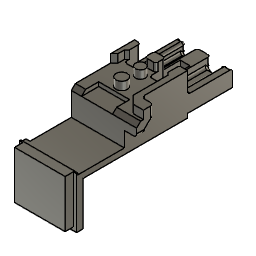
Sony PSP 1000 v29 (Autodesk Fusion 360 design; units mm, degrees)
Autodesk Fusion 360 part; units mm, degrees
sketch "Boceto1" plane through (0, 0, 0) normal (0, 1, 0) x (1, 0, 0)
  line L0 (-3.5, 0) -> (3.5, 0)
  line L1 (3.5, 0) -> (3.5, 6.25)
  line L2 (3.5, 6.25) -> (-3.5, 6.25)
  line L3 (-3.5, 6.25) -> (-3.5, 0)
  line L4 (-2.675, -2.475) -> (-2.675, 0)
  line L5 (2.675, -2.475) -> (2.675, 0)
  circle A0 centre (0, -2.475) radius 2.675
  point P0 (0, -2.475)
  point P1 (2.675, -2.475)
  point P2 (-2.675, -2.475)
  point P3 (0, -5.15)
  dimension "d1" = 7
  dimension "d2" = 3.5
  dimension "d3" = 6.25
  dimension "d43" = 11.4
  dimension "d44" = 2.675
  dimension "d45" = 2.675
  dimension "d46" = 2.675
  dimension "d47" = 2.675
  constraint horizontal L0
  constraint vertical L1
  constraint horizontal L2
  constraint vertical L3
  constraint coincident P2 L4.start
  constraint coincident L0 L4.end
  constraint perpendicular L0 L4
  constraint coincident P1 L5.start
  constraint coincident L0 L5.end
  constraint perpendicular L0 L5
  constraint coincident P0 A0.centre
  constraint coincident P1 A0
  constraint tangent L5 A0
  measures "d1" distance of L1.end L2.end
  measures "d2" distance of origin L0.end
  measures "d3" distance of L0.start L2.end
  measures "d43" vertical distance of L2.end P3
  measures "d44" distance of P0 P3
  measures "d45" horizontal distance of P0 P2
  measures "d46" horizontal distance of P0 P1
  measures "d47" vertical distance of P2 P3
extrude "Extruir13" add sketch "Boceto1" against normal blind 0.5 contours L0 L1 L2 L3 A0
sketch "Boceto10" plane through (0, -0.5, 0) normal (0, -1, 0) x (1, 0, 0)
  line L0 (3.5, 0) -> (1.0149, 0)
  arc A0 (-1.0149, 0) -> (1.0149, 0) centre (0, 2.475) ccw
  line L1 (-1.0149, 0) -> (-3.5, 0)
  line L2 (-3.5, 0) -> (-3.5, -6.25)
  line L3 (-3.5, -6.25) -> (3.5, -6.25)
  line L4 (3.5, -6.25) -> (3.5, 0)
  line L5 (3.1, 0) -> (3.1, -5.85)
  line L6 (3.1, -5.85) -> (-3.1, -5.85)
  line L7 (-3.1, -5.85) -> (-3.1, 0)
  dimension "d50" = 0.4
  dimension "d51" = 0.4
  dimension "d52" = 0.4
  constraint vertical L5
  constraint horizontal L6
  constraint vertical L7
  constraint coincident L1 L7.end
  constraint coincident L0 L5.start
  measures "d50" horizontal distance of L2.end L6.end
  measures "d51" horizontal distance of L3.end L5.end
  measures "d52" vertical distance of L2.end L6.end
extrude "Extruir14" add sketch "Boceto10" along normal blind 1.3 contours L0 A0 L1 L5 L6 L7
extrude "Extruir15" add sketch "Boceto1" against normal blind 1.6 contours L0 L4 A0 | L0 A0 | L0 A0 | L0 L5 A0
sketch "Boceto11" plane through (0, 0, 0) normal (0, 1, 0) x (-1, 0, 0)
  line L0 (-2.675, 0) -> (-3.5, 0)
  line L1 (-3.5, 0) -> (-3.5, -6.25)
  line L2 (-3.5, -6.25) -> (3.5, -6.25)
  line L3 (3.5, -6.25) -> (3.5, 0)
  line L4 (3.5, 0) -> (2.675, 0)
  line L5 (2.675, 0) -> (2.675, 2.475)
  arc A0 (2.675, 2.475) -> (-2.675, 2.475) centre (0, 2.475) ccw
  line L6 (-2.675, 2.475) -> (-2.675, 0)
  line L7 (3.5, -1.5) -> (-3.5, -1.5)
  line L8 (-3.5, -1.5) -> (-3.5, 4.5)
  line L9 (3.5, -1.5) -> (3.5, 4.5)
  line L10 (-3.5, 4.5) -> (3.5, 4.5)
  point P0 (-3.5, -1.5)
  point P1 (3.5, -1.5)
  dimension "d57" = 1.5
  dimension "d58" = 1.5
  dimension "d59" = 6
  dimension "d60" = 6
  constraint coincident L3 P1
  constraint coincident P1 L7.start
  constraint coincident P0 L7.end
  constraint perpendicular L1 L7
  constraint perpendicular L7 L8
  constraint perpendicular L7 L9
  measures "d57" distance of L0.end P0
  measures "d58" distance of L3.end P1
  measures "d59" distance of P0 L8.end
  measures "d60" distance of P1 L9.end
extrude "Extruir16" add sketch "Boceto11" along normal blind 12.8 contours L0 L1 L3 L4 L5 A0 L6 L7 L8 L9 L10 | L0 A0 L6 L8 L10 | A0 L10 | L4 L5 A0 L9 L10
sketch "Boceto12" plane through (0, 12.8, 0) normal (0, 1, 0) x (-1, 0, 0)
  line L0 (3.5, -1.5) -> (3.5, 4.5)
  line L1 (3.5, 4.5) -> (1.7479, 4.5)
  arc A0 (1.7479, 4.5) -> (-1.7479, 4.5) centre (0, 2.475) ccw
  line L2 (-1.7479, 4.5) -> (-3.5, 4.5)
  line L3 (-3.5, 4.5) -> (-3.5, -1.5)
  line L4 (-3.5, -1.5) -> (3.5, -1.5)
  line L5 (1.7479, 4.5) -> (-1.7479, 4.5)
  constraint coincident L1.end A0.start
  constraint coincident A0.end L2.start
extrude "Extruir17" cut sketch "Boceto12" against normal blind 4.5 contours A0 L5
sketch "Boceto13" plane through (0, 0, -1.5) normal (0, 0, -1) x (1, 0, 0)
  line L0 (3.5, 0) -> (-3.5, 0)
  line L1 (-3.5, 0) -> (-3.5, -12.8)
  line L2 (-3.5, -12.8) -> (3.5, -12.8)
  line L3 (3.5, -12.8) -> (3.5, 0)
  line L4 (-3.5, -11.8) -> (2.9, -11.8)
  line L5 (2.9, -11.8) -> (2.9, 0)
  dimension "d65" = 1
  dimension "d66" = 0.6
  constraint coincident L1 L4.start
  constraint perpendicular L1 L4
  constraint coincident L0 L5.end
  constraint perpendicular L0 L5
  measures "d65" distance of L1.end L4.start
  measures "d66" horizontal distance of L2.end L4.end
extrude "Extruir18" cut sketch "Boceto13" against normal blind 0.6 contours L0 L1 L2 L3 L4 L5
sketch "Boceto14" plane through (0, 0, 0) normal (0, -1, 0) x (1, 0, 0)
  line L0 (2.675, 0) -> (3.5, 0)
  line L1 (3.5, 0) -> (3.5, 4.5)
  line L2 (3.5, 4.5) -> (1.7479, 4.5)
  arc A0 (2.675, 2.475) -> (1.7479, 4.5) centre (0, 2.475) ccw
  line L3 (2.675, 2.475) -> (2.675, 0)
  line L4 (3.5, 3.5) -> (1.7479, 4.5)
  dimension "d69" = 1
  constraint coincident L1 L4.start
  constraint coincident L2.end A0.end
  measures "d69" distance of L1.end L4.start
extrude "Extruir20" cut 1 faces at (0.4809, 8.3, 4.5759) along direction (0, -1, 0) blind 15
sketch "Boceto15" plane through (0, 0, 4.5) normal (0, 0, 1) x (-1, 0, 0)
  line L0 (-1.7479, 0) -> (-3.5, 0)
  line L1 (-3.5, 0) -> (-3.5, -12.8)
  line L2 (-3.5, -12.8) -> (3.5, -12.8)
  line L3 (3.5, -12.8) -> (3.5, 0)
  line L4 (3.5, 0) -> (1.7479, 0)
  line L5 (1.7479, 0) -> (1.7479, 1.6)
  line L6 (1.7479, 1.6) -> (-1.7479, 1.6)
  line L7 (-1.7479, 1.6) -> (-1.7479, 0)
  line L8 (3.5, -5.56) -> (-3.5, -5.56)
  dimension "d75" = 5.56
  constraint coincident L3 L8.start
  constraint coincident L1 L8.end
  constraint perpendicular L1 L8
  measures "d75" distance of L3.end L8.start
extrude "Extruir21" cut sketch "Boceto15" against normal blind 4.5 contours L0 L1 L3 L4 L5 L6 L7 L8
extrude "Extruir22" cut 1 faces at (-2.0569, -1.6, 2.325) along direction (0, 1, 0) blind 2.5
extrude "Extruir23" cut 1 faces at (2.0569, -1.6, 2.325) along direction (0, 1, 0) blind 3.5
extrude "Extruir24" cut 1 faces at (1.1667, 7.9733, 4.5) along direction (0, 0, -1) blind 1.35
extrude "Extruir25" add 1 faces at (-1.1667, 5.56, 2.1) along direction (0, -1, 0) blind 0.5
sketch "Boceto16" plane through (0, 0, 3.15) normal (0, 0, 1) x (-1, 0, 0)
  line L0 (-3.5, -5.06) -> (-3.5, -12.8)
  line L1 (-3.5, -12.8) -> (3.5, -12.8)
  line L2 (3.5, -12.8) -> (3.5, -5.06)
  line L3 (2.55, -10.31) -> (2.55, -12.8)
  line L4 (-2.79, -12.8) -> (-2.79, -6.84)
  line L5 (-2.79, -6.84) -> (-3.5, -6.14)
  circle A0 centre (-0.12, -8.11) radius 0.696
  circle A1 centre (-0.12, -10.4) radius 0.6
  line L6 (2.55, -10.31) -> (3.5, -9.38)
  line L7 (1.75, -7.16) -> (-2.05, -7.16)
  line L8 (-2.05, -7.16) -> (-2.05, -5.06)
  line L9 (1.75, -5.06) -> (1.75, -7.16)
  line L10 (3.5, -5.06) -> (-3.5, -5.06)
  point P0 (-0.12, -10.4)
  point P1 (-0.12, -8.11)
  dimension "d7" = 8.325
  dimension "d16" = 2.7
  dimension "d87" = 1.392
  dimension "d88" = 1.2
  dimension "d89" = 2.29
  dimension "d90" = 0.95
  dimension "d91" = 2.49
  dimension "d93" = 0.71
  dimension "d94" = 5.96
  dimension "d95" = 6.66
  dimension "d96" = 3.42
  dimension "d97" = 3.62
  dimension "d98" = 2.4
  dimension "d102" = 2.1
  dimension "d103" = 1.75
  dimension "d104" = 3.8
  constraint coincident L1 L3.end
  constraint perpendicular L1 L3
  constraint coincident L1 L4.start
  constraint perpendicular L1 L4
  constraint coincident L0 L5.end
  constraint coincident P1 A0.centre
  constraint coincident P0 A1.centre
  constraint coincident L2 L6.end
  constraint horizontal L7
  constraint vertical L8
  constraint vertical L9
  constraint coincident L9.start L10
  measures "d87" diameter of A0
  measures "d88" diameter of A1
  measures "d89" distance of P1 P0
  measures "d90" distance of L1.end L3.end
  measures "d91" distance of L3.start L3.end
  measures "d93" distance of L0.end L4.start
  measures "d94" distance of L4.start L4.end
  measures "d95" distance of L0.end L5.end
  measures "d96" distance of L1.end L6.end
  measures "d97" horizontal distance of L1.end P0
  measures "d98" vertical distance of L1.end P0
  measures "d102" distance of L7.start L9.start
  measures "d103" horizontal distance of L2.end L7.start
  measures "d104" distance of L7.start L7.end
chamfer "Chaflán2" distance 0.5 angle 45 1 edges at (0, 5.06, 3.15)
extrude "Extruir26" add sketch "Boceto16" along normal blind 1 contours L0 L1 L4 L5 | L1 L2 L3 L6 | A0 | A1
extrude "Extruir27" cut sketch "Boceto16" against normal blind 0.5 contours L7 L8 L9 L10
sketch "Boceto17" plane through (0, 12.8, 0) normal (0, 1, 0) x (-1, 0, 0)
  line L0 (2.55, 3.15) -> (-2.79, 3.15)
  line L1 (-2.79, 3.15) -> (-2.79, 4.15)
  line L2 (-2.79, 4.15) -> (-3.5, 4.15)
  line L3 (-3.5, 4.15) -> (-3.5, -0.9)
  line L4 (-3.5, -0.9) -> (3.5, -0.9)
  line L5 (3.5, -0.9) -> (3.5, 4.15)
  line L6 (3.5, 4.15) -> (2.55, 4.15)
  line L7 (2.55, 4.15) -> (2.55, 3.15)
  line L8 (-3.5, -0.4) -> (3.5, -0.4)
  line L9 (-3.5, 1.6) -> (3.5, 1.6)
  dimension "d109" = 0.5
  dimension "d110" = 2
  constraint coincident L3 L8.start
  constraint coincident L5 L8.end
  constraint perpendicular L5 L8
  constraint coincident L3 L9.start
  constraint coincident L5 L9.end
  constraint perpendicular L5 L9
  measures "d109" distance of L3.end L8.start
  measures "d110" distance of L8.start L9.start
extrude "Extruir29" add sketch "Boceto17" along normal blind 5.5 contours L3 L5 L8 L9
sketch "Boceto18" plane through (0, 0, 1.6) normal (0, 0, 1) x (-1, 0, 0)
  line L0 (3.5, -12.8) -> (-3.5, -12.8)
  line L1 (-3.5, -12.8) -> (-3.5, -18.3)
  line L2 (-3.5, -18.3) -> (3.5, -18.3)
  line L3 (3.5, -18.3) -> (3.5, -12.8)
  line L4 (-0.6, -13) -> (0.6, -13)
  line L5 (0.6, -13) -> (0.6, -16)
  line L6 (0.6, -16) -> (-0.6, -16)
  line L7 (-0.6, -16) -> (-0.6, -13)
  dimension "d113" = 1.2
  dimension "d114" = 7
  dimension "d115" = 2.9
  dimension "d128" = 0.2
  constraint horizontal L4
  constraint vertical L5
  constraint horizontal L6
  constraint vertical L7
  measures "d113" distance of L5.end L6.end
  measures "d114" distance of L1.end L2.end
  measures "d115" horizontal distance of L1.end L6.end
  measures "d128" vertical distance of L0.end L4.start
extrude "Extruir30" cut sketch "Boceto18" against normal blind 3 contours L4 L5 L6 L7
sketch "Boceto19" plane through (0, 0, 3.15) normal (0, 0, 1) x (-1, 0, 0)
  circle A0 centre (-0.12, -8.11) radius 0.696
  line L0 (1.75, -5.56) -> (1.75, -7.16)
  line L1 (1.75, -7.16) -> (-2.05, -7.16)
  line L2 (-2.05, -7.16) -> (-2.05, -5.56)
  line L3 (-2.05, -5.56) -> (-3.5, -5.56)
  line L4 (-3.5, -5.56) -> (-3.5, -6.14)
  line L5 (-3.5, -6.14) -> (-2.79, -6.84)
  line L6 (-2.79, -6.84) -> (-2.79, -12.8)
  line L7 (-2.79, -12.8) -> (2.55, -12.8)
  line L8 (2.55, -12.8) -> (2.55, -10.31)
  line L9 (2.55, -10.31) -> (3.5, -9.38)
  line L10 (3.5, -9.38) -> (3.5, -5.56)
  line L11 (3.5, -5.56) -> (1.75, -5.56)
  circle A1 centre (-0.12, -10.4) radius 0.6
  line L12 (2.25, -12.8) -> (0.55, -12.8)
  line L13 (0.55, -12.8) -> (0.55, -10.8)
  line L14 (0.55, -10.8) -> (2.25, -10.8)
  line L15 (2.25, -10.8) -> (2.25, -12.8)
  line L16 (-2.49, -12.8) -> (-0.79, -12.8)
  line L17 (-0.79, -12.8) -> (-0.79, -10.8)
  line L18 (-0.79, -10.8) -> (-2.49, -10.8)
  line L19 (-2.49, -10.8) -> (-2.49, -12.8)
  dimension "d118" = 1.7
  dimension "d119" = 1.7
  dimension "d120" = 0.3
  dimension "d121" = 0.3
  dimension "d122" = 2
  dimension "d123" = 2
  constraint horizontal L12
  constraint vertical L13
  constraint horizontal L14
  constraint vertical L15
  constraint coincident L7 L12.start
  constraint horizontal L16
  constraint vertical L17
  constraint horizontal L18
  constraint vertical L19
  constraint coincident L7 L16.start
  measures "d118" distance of L12.start L12.end
  measures "d119" distance of L16.start L16.end
  measures "d120" distance of L7.end L12.start
  measures "d121" distance of L6.end L16.start
  measures "d122" distance of L12.end L13.end
  measures "d123" distance of L16.end L17.end
extrude "Extruir31" cut sketch "Boceto19" against normal blind 1.55 contours L7 L12 L13 L14 L15 | L7 L16 L17 L18 L19
sketch "Boceto20" plane through (-3.5, 0, 0) normal (-1, 0, 0) x (0, -1, 0)
  line L0 (-5.06, 2.65) -> (-5.56, 3.15)
  line L1 (-5.56, 3.15) -> (-9.38, 3.15)
  line L2 (-9.38, 3.15) -> (-9.38, 4.15)
  line L3 (-9.38, 4.15) -> (-12.8, 4.15)
  line L4 (-12.8, 4.15) -> (-12.8, 1.6)
  line L5 (-12.8, 1.6) -> (-18.3, 1.6)
  line L6 (-18.3, 1.6) -> (-18.3, -0.4)
  line L7 (-18.3, -0.4) -> (-12.8, -0.4)
  line L8 (-12.8, -0.4) -> (-12.8, -0.9)
  line L9 (-12.8, -0.9) -> (-11.8, -0.9)
  line L10 (-11.8, -0.9) -> (-11.8, -1.5)
  line L11 (-11.8, -1.5) -> (0, -1.5)
  line L12 (0, -1.5) -> (0, -6.25)
  line L13 (0, -6.25) -> (0.5, -6.25)
  line L14 (0.5, -6.25) -> (0.5, 0)
  line L15 (0.5, 0) -> (-5.06, 0)
  line L16 (-5.06, 0) -> (-5.06, 2.65)
  line L17 (0, -1.5) -> (0, 0)
  constraint coincident L11.end L12.start
  constraint coincident L17.end origin
extrude "Extruir32" cut sketch "Boceto20" against normal blind 0.5 contours L0 L1 L2 L3 L4 L5 L6 L7 L8 L9 L10 L11 L15 L16 L17
extrude "Extruir33" add 1 faces at (-1.0333, -0.5, -6.1167) along direction (0, -1, 0) blind 0.3
sketch "Boceto21" plane through (0, 0, 0) normal (0, 0, 1) x (-1, 0, 0)
  line L0 (3, -5.06) -> (3, 0)
  line L1 (3, 0) -> (3.5, 0)
  line L2 (3.5, 0) -> (3.5, 0.8)
  line L3 (3.5, 0.8) -> (3.1, 0.8)
  line L4 (3.1, 0.8) -> (3.1, 1.8)
  line L5 (3.1, 1.8) -> (1.0149, 1.8)
  line L6 (1.0149, 1.8) -> (1.0149, 1.6)
  line L7 (1.0149, 1.6) -> (-1.0149, 1.6)
  line L8 (-1.0149, 1.6) -> (-1.0149, 1.8)
  line L9 (-1.0149, 1.8) -> (-3.1, 1.8)
  line L10 (-3.1, 1.8) -> (-3.1, 0.8)
  line L11 (-3.1, 0.8) -> (-3.5, 0.8)
  line L12 (-3.5, 0.8) -> (-3.5, -5.06)
  line L13 (-3.5, -5.06) -> (3, -5.06)
  line L14 (-3.1, 0.64) -> (3.1, 0.64)
  line L15 (3.1, 0.64) -> (3.5, 0.64)
  line L16 (-3.1, 0.64) -> (-3.5, 0.64)
  dimension "d133" = 1.16
  constraint coincident L10 L14.start
  constraint coincident L4 L14.end
  constraint perpendicular L4 L14
  constraint coincident L2 L15.end
  constraint perpendicular L2 L15
  constraint coincident L12 L16.end
  constraint perpendicular L12 L16
  measures "d133" distance of L4.end L14.end
extrude "Extruir34" cut sketch "Boceto21" against normal blind 0.2 contours L0 L1 L2 L12 L13 L14 L15 L16
extrude "Extruir35" add 1 faces at (-0.2287, -1.6, -0.0368) along direction (0, -1, 0) blind 0.2
sketch "Boceto22" plane through (0, 0, 3.15) normal (0, 0, 1) x (-1, 0, 0)
  line L0 (3, -9.8695) -> (3, -5.56)
  line L1 (3, -5.56) -> (1.75, -5.56)
  line L2 (1.75, -5.56) -> (1.75, -7.16)
  line L3 (1.75, -7.16) -> (-2.05, -7.16)
  line L4 (-2.05, -7.16) -> (-2.05, -5.56)
  line L5 (-2.05, -5.56) -> (-3.5, -5.56)
  line L6 (-3.5, -5.56) -> (-3.5, -6.14)
  line L7 (-3.5, -6.14) -> (-2.79, -6.84)
  line L8 (-2.79, -6.84) -> (-2.79, -12.8)
  line L9 (-2.79, -12.8) -> (-2.49, -12.8)
  line L10 (-2.49, -12.8) -> (-2.49, -10.8)
  line L11 (-2.49, -10.8) -> (-0.79, -10.8)
  line L12 (-0.79, -10.8) -> (-0.79, -12.8)
  line L13 (-0.79, -12.8) -> (0.55, -12.8)
  line L14 (0.55, -12.8) -> (0.55, -10.8)
  line L15 (0.55, -10.8) -> (2.25, -10.8)
  line L16 (2.25, -10.8) -> (2.25, -12.8)
  line L17 (2.25, -12.8) -> (2.55, -12.8)
  line L18 (2.55, -12.8) -> (2.55, -10.31)
  line L19 (2.55, -10.31) -> (3, -9.8695)
  circle A0 centre (-0.12, -8.11) radius 0.696
  circle A1 centre (-0.12, -10.4) radius 0.6
  line L20 (-0.79, -11.6) -> (0.55, -11.6)
  line L21 (-2.49, -11.4) -> (-2.79, -11.4)
  line L22 (2.25, -11.4) -> (2.55, -11.4)
  dimension "d136" = 0.8
  dimension "d142" = 0.6
  dimension "d143" = 0.6
  constraint coincident L12 L20.start
  constraint coincident L14 L20.end
  constraint perpendicular L14 L20
  constraint coincident L8 L21.end
  constraint perpendicular L8 L21
  constraint coincident L18 L22.end
  constraint perpendicular L18 L22
  constraint coincident L10 L21.start
  constraint coincident L16 L22.start
  measures "d136" distance of L14.end L20.end
  measures "d142" distance of L10.end L21.start
  measures "d143" distance of L15.end L22.start
extrude "Extruir36" add sketch "Boceto22" along normal blind 1 contours L16 L17 L18 L22 | L12 L13 L14 L20 | L8 L9 L10 L21
fillet "Empalme1" radius 0.3 2 edges at (-0.55, 11.6, 3.65) (0.79, 11.6, 3.65)
chamfer "Chaflán3" distance 0.3 angle 45 2 edges at (2.79, 11.4, 3.65) (-2.55, 11.4, 3.65)
sketch "Boceto23" plane through (3.5, 0, 0) normal (1, 0, 0) x (0, 1, 0)
  line L0 (5.06, 2.65) -> (5.06, -0.2)
  line L1 (5.06, -0.2) -> (-0.64, -0.2)
  line L2 (-0.8, 0) -> (-0.8, -6.25)
  line L3 (-0.8, -6.25) -> (0, -6.25)
  line L4 (0, -6.25) -> (0, -0.9)
  line L5 (0, -0.9) -> (12.8, -0.9)
  line L6 (12.8, -0.9) -> (12.8, -0.4)
  line L7 (12.8, -0.4) -> (18.3, -0.4)
  line L8 (18.3, -0.4) -> (18.3, 1.6)
  line L9 (18.3, 1.6) -> (12.8, 1.6)
  line L10 (12.8, 1.6) -> (12.8, 4.15)
  line L11 (12.8, 4.15) -> (6.14, 4.15)
  line L12 (6.14, 4.15) -> (6.14, 3.15)
  line L13 (6.14, 3.15) -> (5.56, 3.15)
  line L14 (5.56, 3.15) -> (5.06, 2.65)
  line L15 (5.06, 1.65) -> (7.14, 1.65)
  line L16 (7.14, 1.65) -> (7.14, 4.15)
  line L17 (-0.64, -0.2) -> (-0.64, 0)
  line L18 (-0.64, 0) -> (-0.8, 0)
  dimension "d144" = 1
  dimension "d145" = 2.5
  constraint coincident L0 L15.start
  constraint perpendicular L0 L15
  constraint coincident L11 L16.end
  constraint perpendicular L11 L16
  measures "d144" distance of L11.end L16.end
  measures "d145" distance of L15.end L16.end
extrude "Extruir37" add sketch "Boceto23" along normal blind 1.5 contours L0 L11 L12 L13 L14 L15 L16
chamfer "Chaflán4" distance 1 angle 45 1 edges at (4.25, 7.14, 1.65)
fillet "Empalme2" radius 0.4 6 edges at (5, 5.6, 1.65) (5, 6.64, 2.15) (5, 7.14, 3.4) (3.5, 7.14, 3.4) (4.25, 7.14, 2.65) (4.25, 6.14, 1.65)
sketch "Boceto24" plane through (0, 0, 1.6) normal (0, 0, 1) x (-1, 0, 0)
  line L0 (3, -18.3) -> (3, -12.8)
  line L1 (3, -12.8) -> (2.25, -12.8)
  line L2 (2.25, -12.8) -> (2.25, -10.8)
  line L3 (2.25, -10.8) -> (0.55, -10.8)
  line L4 (0.55, -10.8) -> (0.55, -12.8)
  line L5 (0.55, -12.8) -> (-0.79, -12.8)
  line L6 (-0.79, -12.8) -> (-0.79, -10.8)
  line L7 (-0.79, -10.8) -> (-2.49, -10.8)
  line L8 (-2.49, -10.8) -> (-2.49, -12.8)
  line L9 (-2.49, -12.8) -> (-3.5, -12.8)
  line L10 (-3.5, -12.8) -> (-3.5, -18.3)
  line L11 (-3.5, -18.3) -> (3, -18.3)
  line L12 (0.6, -13) -> (0.6, -16)
  line L13 (0.6, -16) -> (-0.6, -16)
  line L14 (-0.6, -16) -> (-0.6, -13)
  line L15 (-0.6, -13) -> (0.6, -13)
  line L16 (-2.49, -12.8) -> (-2.49, -18.3)
  line L17 (-0.79, -12.8) -> (-0.79, -18.3)
  line L18 (2.25, -12.8) -> (2.25, -18.3)
  line L19 (0.8, -12.824) -> (0.8, -18.3)
  line L20 (0.55, -12.3571) -> (0.8, -12.824)
  dimension "d151" = 0.2
  constraint coincident L8.end L9.start
  constraint coincident L11 L16.end
  constraint perpendicular L11 L16
  constraint coincident L5.end L6.start
  constraint coincident L11 L17.end
  constraint perpendicular L11 L17
  constraint coincident L1.end L2.start
  constraint coincident L11 L18.end
  constraint perpendicular L11 L18
  constraint coincident L11 L19.end
  constraint perpendicular L11 L19
  constraint coincident L4 L20.start
  measures "d151" horizontal distance of L12.end L19.end
extrude "Extruir38" cut sketch "Boceto24" against normal blind 1 contours L2 L3 L4 L11 L18 L19 L20 | L6 L7 L8 L11 L16 L17
chamfer "Chaflán5" distance 0.7 angle 45 2 edges at (-1.525, 18.3, 0.6) (1.64, 18.3, 0.6)
fillet "Empalme3" radius 0.3 32 edges at (2.49, 14.2, 0.6) (1.64, 10.8, 0.6) (0.79, 14.2, 0.6) (-0.8, 15.212, 0.6) (-0.675, 12.5906, 0.6) (-0.55, 11.5785, 0.6) (-2.25, 14.2, 0.6) (2.49, 17.95, 0.25) (0.79, 17.95, 0.25) (-0.8, 17.95, 0.25) (-2.25, 17.95, 0.25) (2.49, 15.55, 1.6) (-2.25, 15.55, 1.6) (-2.25, 18.3, 0.75) (2.49, 18.3, 0.75) (0.79, 18.3, 0.75) (-0.8, 18.3, 0.75) (0.79, 10.8, 1.875) (2.49, 10.8, 1.875) (-0.55, 10.8, 1.875) (-2.25, 10.8, 1.875) (-0.55, 12.8, 2.875) (0.79, 12.8, 2.875) (2.49, 12.8, 2.875) (-2.25, 12.8, 2.875) (2.995, 12.8, 1.6) (-2.625, 12.8, 1.6) (-2.625, 18.3, 1.6) (2.995, 18.3, 1.6) (-0.05, 11.8, -1.5) (-1.525, 18.3, -0.1) (1.64, 18.3, -0.1)
extrude "Extruir39" add 1 faces at (4, 6.14, 3.8167) along direction (0, -1, 0) blind 0.25
sketch "Boceto25" plane through (0, 0, 4.15) normal (0, 0, 1) x (-1, 0, 0)
  arc A0 (-2.79, -12.8) -> (-2.49, -12.5) centre (-2.79, -12.5) ccw
  line L0 (-2.49, -12.5) -> (-2.49, -11.4)
  line L1 (-2.49, -11.4) -> (-2.79, -11.1)
  line L2 (-2.79, -11.1) -> (-2.79, -6.84)
  line L3 (-2.79, -6.84) -> (-3.5, -6.14)
  line L4 (-3.5, -6.14) -> (-3.5, -5.89)
  line L5 (-3.5, -5.89) -> (-5, -5.89)
  line L6 (-5, -5.89) -> (-5, -6.74)
  arc A1 (-5, -6.74) -> (-4.6, -7.14) centre (-4.6, -6.74) ccw
  line L7 (-4.6, -7.14) -> (-3.9, -7.14)
  arc A2 (-3.5, -7.54) -> (-3.9, -7.14) centre (-3.9, -7.54) ccw
  line L8 (-3.5, -7.54) -> (-3.5, -12.8)
  line L9 (-3.5, -12.8) -> (-2.79, -12.8)
  line L10 (-3.5, -6.14) -> (-3.7536, -5.89)
  constraint coincident L3.end L4.start
  constraint coincident L5 L10.end
  constraint parallel L3 L10
extrude "Extruir40" cut sketch "Boceto25" against normal blind 1 contours L4 L5 L10
other "Elemento de malla base8"
equation "d2 = d1 / 2"
equation "d4 = 5.35 mm"
equation "d7 = 11 mm - ( d4 / 2 )"
equation "d8 = 5.4 mm"
equation "d16 = d8 / 2"
equation "d44 = ( 5.35 / 2 ) * 1 mm"
equation "d45 = d44"
equation "d46 = d44"
equation "d47 = d44"
equation "d51 = d50"
equation "d52 = d50"
equation "d58 = d57"
equation "d60 = d59"
equation "d75 = 5.3 mm - 0.5 mm + 0.76 mm"
equation "d87 = 1.9 mm - 0.508 mm"
equation "d91 = 3.25 mm - 0.76 mm"
equation "d94 = 6.72 mm - 0.76 mm"
equation "d95 = 7.42 mm - 0.76 mm"
equation "d96 = 4.18 mm - 0.76 mm"
equation "d115 = d114 / 2 - ( d113 / 2 )"
equation "d119 = d118"
equation "d121 = d120"
equation "d123 = d122"
equation "d133 = 0.4 mm + 0.76 mm"
equation "d143 = d142"
